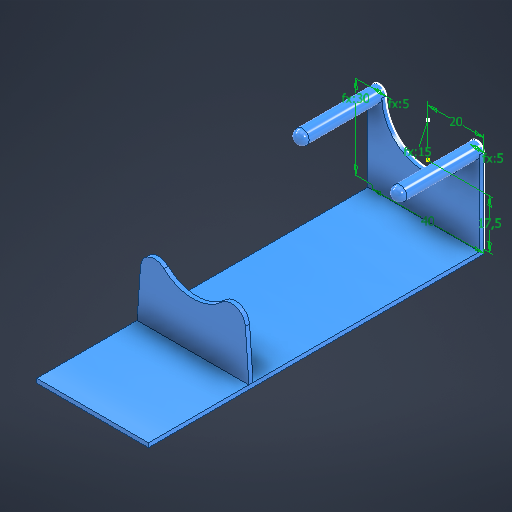
# Autodesk Inventor part: my_portafilter_holder_23ipt
Saved by Autodesk Inventor 2026 (Build 300175000, 175)
## iProperties
Created: 2025-04-17
Part Number: my_portafilter_holder_23ipt
Material: Generic
Document SubType Name: Modeling
Designer: Paul Juschitz
Density: 1 g/cm^3
Appearance: Cyan
Author: Paul Juschitz
Autodesk Inventor part; units mm, degrees
ref_plane "YZ Plane" through (0, 0, 0) normal (1, 0, 0) x (0, 1, 0)
ref_plane "XZ Plane" through (0, 0, 0) normal (0, 1, 0) x (-1, 0, 0)
ref_plane "XY Plane" through (0, 0, 0) normal (0, 0, 1) x (1, 0, 0)
sketch "Sketch1" plane through (0, 0, 0) normal (0, 0, 1) x (1, 0, 0)
  line L0 (20, 12.5) -> (20, -17.5)
  line L1 (20, -17.5) -> (-20, -17.5)
  line L2 (-20, -17.5) -> (-20, 12.5)
  circle A0 centre (-17.5, 12.5) radius 2.5
  circle A1 centre (17.5, 12.5) radius 2.5
  arc A2 (-15, 12.5) -> (15, 12.5) centre (0, 12.5) ccw
  point P0 (0, 0)
  dimension "d0" = 40
  dimension "d2" = 5
  dimension "d3" = 5
  dimension "d4" = 30
  dimension "d5" = 20
  dimension "d6" = 17.5
  dimension "d7" = 15
  constraints: 6 end point, 6 point on circle, 4 tangent, 3 centre point, 1 horizontal, 1 horizontal alignment, 1 parallel, 1 perpendicular
  measures "d0" distance of L0.end L1.end
  measures "d2" diameter of A0
  measures "d3" diameter of A1
  measures "d4" distance of L1.end L2.end
  measures "d5" distance from line of point (0, 0) L0
  measures "d6" distance from line of point (0, 0) L1
  measures "d7" radius of A2
extrude "Extrusion1" add sketch "Sketch1" along normal blind 1.5 contours L0 L1 L2 A0 A2 A1
extrude "Extrusion2" add sketch "Sketch1" along normal blind 30 contours A1 | A0
fillet "Fillet1" radius 2.5 2 edges at (-20, 12.5, 30) (15, 12.5, 30)
sketch "Sketch2" plane through (0, 0, 0) normal (0, 0, 1) x (1, 0, 0)
  line L0 (-20, -17.5) -> (20, -17.5) projected
  line L1 (-20, -17.5) -> (20, -17.5) projected
  line L2 (-20, -17.5) -> (20, -17.5)
  line L3 (20, -17.5) -> (20, -19)
  line L4 (20, -19) -> (-20, -19)
  line L5 (-20, -19) -> (-20, -17.5)
  point P0 (0, 0)
  dimension "d13" = 1.5
  constraints: 8 end point, 3 perpendicular, 1 collinear
  measures "d13" distance of L4.end L0.start
extrude "Extrusion3" add sketch "Sketch2" along normal blind 120
sketch "Sketch5" plane through (-20, -17.5, 1.5) normal (0, 1, 0) x (1, 0, 0)
  line L0 (0, 0) -> (0, -118.5) projected
  line L1 (40, 0) -> (40, -118.5) projected
  line L2 (0, -81.0917) -> (40, -81.0917)
  line L3 (40, -81.0917) -> (40, -82.5917)
  line L4 (40, -82.5917) -> (0, -82.5917)
  line L5 (0, -82.5917) -> (0, -81.0917)
  line L6 (0, 0) -> (40, 0) projected
  point P0 (20, 1.5)
  point P1 (0, -82.5917)
  dimension "d25" = 1.5
  dimension "d26" = 81.0917
  constraints: 8 end point, 2 parallel, 2 point on line, 1 horizontal, 1 perpendicular
  measures "d25" distance between parallel lines of L4 L2
  measures "d26" distance between parallel lines of L6 L2
extrude "Extrusion5" add sketch "Sketch5" along normal blind 40 contours L2 L1 L4 L0
sketch "Sketch7" plane through (-20, -17.5, 84.0917) normal (0, 0, 1) x (1, 0, 0)
  arc A0 (9.6688, 20.825) -> (30.3312, 20.825) centre (20, 31.7) ccw
  line L0 (40, 0) -> (0, 0) projected
  line L1 (40, 0) -> (0, 0)
  line L2 (0, 0) -> (1.2374, 17.5516)
  arc A1 (9.6688, 20.825) -> (1.2374, 17.5516) centre (6.225, 17.2) ccw
  line L3 (40, 0) -> (38.7626, 17.5516)
  arc A2 (38.7626, 17.5516) -> (30.3312, 20.825) centre (33.775, 17.2) ccw
  line L4 (20, 0.597) -> (20, 58.4364) construction
  line L5 (40, 0) -> (40, 40) projected
  line L6 (40, 0) -> (40, 40)
  line L7 (0, 0) -> (0, 40) projected
  line L8 (40, 40) -> (0, 40)
  line L9 (0, 40) -> (0, 0)
  point P0 (20, 17.5)
  dimension "d36" = 30
  dimension "d37" = 31.7
  dimension "d38" = 5
  dimension "d39" = 17.2
  constraints: 14 end point, 6 point on circle, 4 tangent, 3 centre point, 3 vertical, 1 collinear, 1 equal radius, 1 horizontal alignment, 1 perpendicular, 1 point on line, 1 symmetric about line
  measures "d36" diameter of A0
  measures "d37" distance from line of A0.centre L0
  measures "d38" radius of A2
  measures "d39" distance from line of L0 A2.centre
extrude "Extrusion7" cut sketch "Sketch7" against normal up to surface (1.5 mm away) contours A1 L2 L7 L8 L5 L3 A2 A0
equation "\"d2\" = arm_thickness"
equation "\"d3\" = arm_thickness"
equation "\"d4\" = top_prong_height"
equation "\"d7\" = 3 * arm_thickness"
equation "\"d8\" = material_thickness"
equation "\"d10\" = arm_length"
equation "\"d12\" = 0.5 * arm_thickness"
equation "\"d13\" = material_thickness"
equation "\"d25\" = material_thickness"
equation "\"d36\" = handle_cutout_radius"
equation "\"d37\" = top_prong_height + prong_handle_height"
equation "\"arm_thickness\" = 5"
equation "\"material_thickness\" = 1.5"
equation "\"arm_length\" = 30"
equation "\"top_prong_height\" = 30"
equation "\"handle_cutout_radius\" = 30"
equation "\"prong_handle_height\" = 1.7"
body "Solid1"
